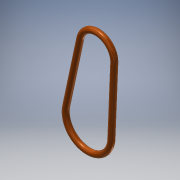
# Autodesk Inventor part: Pulley_Belt
Saved by Autodesk Inventor 2019 (Build 230136000, 136)
## iProperties
Created: 2021-02-23
Part Number: Pulley_Belt
Material: Rubber, Silicone
Document SubType Name: Modeling
Designer: zhanb
Density: 1.25 g/cm^3
Appearance: Smooth - Light Orange
Author: zhanb
Autodesk Inventor part; units mm, degrees
ref_plane "YZ Plane" through (0, 0, 0) normal (1, 0, 0) x (0, 1, 0)
ref_plane "XZ Plane" through (0, 0, 0) normal (0, 1, 0) x (-1, 0, 0)
ref_plane "XY Plane" through (0, 0, 0) normal (0, 0, 1) x (1, 0, 0)
sketch "Sketch1" plane through (0, 0, 0) normal (0, 0, 1) x (1, 0, 0)
  circle A0 centre (0, 0) radius 2.54 construction
  circle A1 centre (-4.787571, -37.499034) radius 13.50645 construction
  circle A2 centre (0, 0) radius 10.33145 construction
  arc A3 (9.516237, -0.408485) -> (-9.313612, 1.995557) centre (0, 0) ccw
  arc A4 (-17.205721, -34.838292) -> (7.900745, -38.04368) centre (-4.787571, -37.499034) ccw
  line L0 (-9.313612, 1.995557) -> (-17.205721, -34.838292)
  line L1 (7.900745, -38.04368) -> (9.516237, -0.408485)
  point P0 (0, 0)
  dimension "d0" = 12.7
  dimension "d1" = 9.525
  constraints: 4 end point, 4 point on circle, 4 tangent, 2 centre point, 1 coincident, 1 concentric
  measures "d0" radius of A4
  measures "d1" radius of A3
sketch "Sketch2" plane through (0, 0, 0) normal (0, 1, 0) x (-1, 0, 0)
  circle A0 centre (-9.516237, 0) radius 1.5875
  point P0 (0, 0)
  dimension "d2" = 3.175
  constraints: 1 centre point, 1 coincident
  measures "d2" diameter of A0
sweep "Sweep1" add profiles "Sketch2" path "Sketch1"
body "Solid1"
